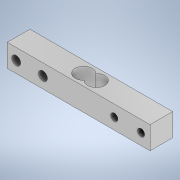
# Autodesk Inventor part: [한진데이타]_4선식_저가형_로드셀_5Kg
Saved by Autodesk Inventor 2021 (Build 250183000, 183)
## iProperties
Created: 2021-01-21
Part Number: [한진데이타]_4선식_저가형_로드셀_5Kg
Material: 알루미늄 6061
Document SubType Name: Modeling
Designer: leejun
Density: 2.7 g/cm^3
Appearance: 알루미늄 - 짙음
Author: leejun
Autodesk Inventor part; units mm, degrees
ref_plane "YZ Plane" through (0, 0, 0) normal (1, 0, 0) x (0, 1, 0)
ref_plane "XZ Plane" through (0, 0, 0) normal (0, 1, 0) x (-1, 0, 0)
ref_plane "XY Plane" through (0, 0, 0) normal (0, 0, 1) x (1, 0, 0)
sketch "스케치1" plane through (0, 0, 0) normal (0, 0, 1) x (1, 0, 0)
  line L0 (0, 0) -> (80, 0)
  line L1 (80, 0) -> (80, 12.7)
  line L2 (80, 12.7) -> (0, 12.7)
  line L3 (0, 12.7) -> (0, 0)
  circle A0 centre (5, 6.35) radius 2.5
  circle A1 centre (20, 6.35) radius 2.5
  circle A2 centre (60, 6.35) radius 2
  circle A3 centre (75, 6.35) radius 2
  circle A4 centre (5, 6.35) radius 6.35 construction
  dimension "d0" = 80
  dimension "d1" = 12.7
  dimension "d2" = 5
  dimension "d3" = 15
  dimension "d4" = 5
  dimension "d5" = 5
  dimension "d6" = 15
  dimension "d7" = 4
  constraints: 8 end point, 5 centre point, 3 horizontal alignment, 2 equal radius, 2 parallel, 2 tangent, 1 coincident, 1 horizontal, 1 perpendicular
  measures "d0" distance of L1.end L2.end
  measures "d1" distance of L2.end L0.start
  measures "d2" distance from line of L3 A0.centre
  measures "d3" distance of A1.centre A0.centre
  measures "d4" diameter of A0
  measures "d5" distance from line of L1 A3.centre
  measures "d6" distance of A3.centre A2.centre
  measures "d7" diameter of A3
extrude "돌출1" add sketch "스케치1" against normal blind 12.7
sketch "스케치2" plane through (0, 12.7, 0) normal (0, 1, 0) x (1, 0, 0)
  circle A0 centre (36.5, 6.35) radius 4.85
  circle A1 centre (43.5, 6.35) radius 4.85
  circle A2 centre (36.5, 6.35) radius 6.35 construction
  line L0 (80, 12.7) -> (0, 12.7) projected
  line L1 (80, 0) -> (0, 0) projected
  circle A3 centre (40, 6.35) radius 3.5 construction
  circle A4 centre (40, 6.35) radius 40 construction
  line L2 (80, 0) -> (80, 12.7) projected
  line L3 (0, 0) -> (0, 12.7) projected
  point P0 (40, 9.7075)
  point P1 (40, 2.9925)
  dimension "d10" = 1.5
  dimension "d11" = 7
  constraints: 5 centre point, 4 tangent, 2 coincident, 2 horizontal alignment, 2 point on circle, 1 equal radius
  measures "d10" radial gap between concentric circles of A2 A0
  measures "d11" distance of A1.centre A0.centre
extrude "돌출2" cut sketch "스케치2" against normal through all contours A0 A1 | A0 A1 | A1 A0
thread "스레드1" size "M5x0.8" class "6H" standard "ANSI Metric M Profile" full length
thread "스레드2" size "M5x0.8" class "6H" standard "ANSI Metric M Profile" full length
thread "스레드3" size "M4x0.7" class "6H" standard "ANSI Metric M Profile" full length
thread "스레드4" size "M4x0.7" class "6H" standard "ANSI Metric M Profile" full length
